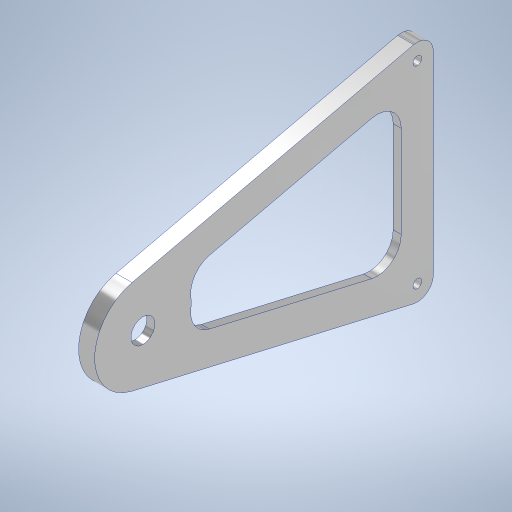
# Autodesk Inventor part: Frame (Motor Side)
Saved by Autodesk Inventor 2023.2 (Build 272271000, 271)
## iProperties
Created: 2022-05-22
Part Number: Frame (Motor Side)
Material: Aluminum 6061
Document SubType Name: Modeling
Designer: Nathan Cai
Density: 2.7 g/cm^3
Appearance: Aluminum - Flat
Mass: 63.0203 g
Surface Area: 136.097 cm^2
Volume: 23.3409 cm^3
Leg_Mounts: 0.625 in
Leg_Offset: 0.750 in
C2C: 4.265 in
Author: Nathan Cai
Autodesk Inventor part; units mm, degrees
ref_plane "YZ Plane" through (0, 0, 0) normal (1, 0, 0) x (0, 1, 0)
ref_plane "XZ Plane" through (0, 0, 0) normal (0, 1, 0) x (-1, 0, 0)
ref_plane "XY Plane" through (0, 0, 0) normal (0, 0, 1) x (1, 0, 0)
sketch "Sketch1" plane through (0, 0, 0) normal (1, 0, 0) x (0, 1, 0)
  circle A0 centre (0, 0) radius 4.7625 construction
  line L0 (0, 0) -> (0, 108.331) construction
  circle A1 centre (0, 108.331) radius 4.7625
  circle A2 centre (0, 108.331) radius 76.2 construction
  circle A3 centre (0, 108.331) radius 19.05
  line L1 (0, 0) -> (38.1, 0) construction
  circle A4 centre (38.1, 0) radius 1.7526
  circle A5 centre (38.1, 0) radius 6.35
  line L2 (18.5597, 112.6252) -> (44.2866, 1.4314)
  line L3 (10.2351, 92.2641) -> (31.9134, -1.4314)
  circle A6 centre (-38.1, 0) radius 1.7526
  circle A7 centre (-38.1, 0) radius 6.35
  line L4 (-18.5597, 112.6252) -> (-44.2866, 1.4314)
  line L5 (-10.2351, 92.2641) -> (-31.9134, -1.4314)
  line L6 (38.1, 6.35) -> (-38.1, 6.35)
  line L7 (-38.1, -6.35) -> (38.1, -6.35)
  line L8 (38.1, 0) -> (15.5738, 97.3602) construction
  circle A8 centre (19.05, 82.3358) radius 1.7526
  circle A9 centre (-19.05, 82.3358) radius 1.7526
  line L9 (19.05, 82.3358) -> (-19.05, 82.3358) construction
  circle A10 centre (15.875, 82.3358) radius 6.35
  circle A11 centre (15.875, 82.3358) radius 1.7526
  circle A12 centre (-15.875, 82.3358) radius 6.35
  circle A13 centre (-15.875, 82.3358) radius 1.7526
  arc A14 (31.7424, -0.6924) -> (-31.1085, -6.35) centre (0, 0) ccw construction
  arc A15 (44.45, 0) -> (-44.45, 0) centre (0, 0) ccw construction
  point P0 (44.2067, -1.741)
  point P1 (-22.5544, 39.0194)
  point P2 (-10.2351, 92.2641)
  point P3 (30.1131, 6.35)
  point P4 (-30.1131, 6.35)
  point P5 (-13.9309, 76.2907)
  point P6 (-11.4733, 86.9126)
  point P7 (11.4733, 86.9126)
  point P8 (13.9309, 76.2907)
  point P9 (22.7465, 38.189)
  point P10 (-22.7465, 38.189)
  point P11 (-40.2576, 18.8447)
  point P12 (-44.3636, 7.3939)
  point P13 (-31.75, 0)
  point P14 (31.75, 0)
  point P15 (44.3636, 7.3939)
  point P16 (40.2576, 18.8447)
  point P17 (-28.2125, 14.5642)
  point P18 (31.8736, 5.0775)
  point P19 (-31.7424, -0.6924)
  point P20 (28.2125, 14.5642)
  dimension "d0" = 9.525
  dimension "C2C" = 108.331
  dimension "d3" = 9.525
  dimension "d4" = 152.4
  dimension "d5" = 38.1
  dimension "d6" = 38.1
  dimension "d7" = 3.5052
  dimension "d8" = 12.7
  dimension "d9" = 0
  dimension "d10" = 12.7
  dimension "d37" = 3.5052
  dimension "Leg_Offset" = 19.05
  dimension "d39" = 12.7
  dimension "d40" = 3.5052
  dimension "Leg_Mounts" = 15.875
  dimension "d42" = 12.7
  constraints: 20 end point, 18 point on circle, 16 centre point, 11 coincident, 10 symmetric about line, 7 tangent, 6 point on line, 2 horizontal, 2 parallel, 1 vertical, 5 other
  measures "d0" diameter of A0
  measures "C2C" distance of L0.start L0.end
  measures "d3" diameter of A1
  measures "d4" diameter of A2
  measures "d5" diameter of A3
  measures "d6" distance of L1.start L1.end
  measures "d7" diameter of A4
  measures "d8" diameter of A5
  measures "d9" distance from line of A0.centre L1
  measures "d10" distance between parallel lines of L2 L3
  measures "d37" diameter of A8
  measures "Leg_Offset" distance from line of L0 L9.start
  measures "d39" diameter of A10
  measures "d40" diameter of A11
  measures "Leg_Mounts" distance from line of L0 A11.centre
  measures "d42" radial gap between concentric circles of A14 A15
extrude "Extrusion1" add sketch "Sketch1" along normal blind 6.35 contours A3 | A3 L2 A5 L6 L3 A10 | A3 L5 A12 L6 A7 L4 | A5 | A10 L3 | A7 | A5 L3 L6 | L5 A12 | L6 L5 A7 | A7 L5 L6 L3 A5 L7 | A8 A11 | A11 A8 | A8 A11 | A9 A13 | A9 A13 | A13 A9 picked at (13.1931, 81.7042) picked at (-13.1931, 81.7042)
fillet "Fillet1" radius 9.525 4 edges at (3.175, 10.2351, 92.2641) (3.175, -10.2351, 92.2641) (3.175, 30.1131, 6.35) (3.175, -30.1131, 6.35)
sketch "Sketch2" plane through (0, 0, 0) normal (1, 0, 0) x (0, 0, -1)
  line L0 (-1.4314, 44.2866) -> (-112.6252, 18.5597) projected
  circle A0 centre (0, 38.1) radius 6.35
  circle A1 centre (0, -38.1) radius 1.7526 projected
  arc A2 (-1.4314, -44.2866) -> (6.35, -38.1) centre (0, -38.1) ccw projected
  circle A3 centre (0, -38.1) radius 6.35
  circle A4 centre (0, 38.1) radius 1.7526 projected
  line L1 (-18.0221, -27.4125) -> (-82.0952, -12.5879) projected
  circle A5 centre (0, -38.1) radius 1.7526 projected
  circle A6 centre (-108.331, 0) radius 4.7625 projected
  circle A7 centre (0, 38.1) radius 1.7526 projected
  line L2 (6.35, -38.1) -> (6.35, 38.1) projected
  arc A8 (6.35, 38.1) -> (-1.4314, 44.2866) centre (0, 38.1) ccw projected
  line L3 (-1.4314, 44.2866) -> (-112.6252, 18.5597) projected
  line L4 (-112.6252, -18.5597) -> (-1.4314, -44.2866) projected
  arc A9 (-1.4314, -44.2866) -> (6.35, -38.1) centre (0, -38.1) ccw projected
  line L5 (-18.0221, -27.4125) -> (-82.0952, -12.5879) projected
  circle A10 centre (0, -38.1) radius 1.7526 projected
  circle A11 centre (-108.331, 0) radius 4.7625 projected
  circle A12 centre (0, 38.1) radius 1.7526 projected
  line L6 (6.35, -38.1) -> (6.35, 38.1) projected
  arc A13 (6.35, 38.1) -> (-1.4314, 44.2866) centre (0, 38.1) ccw projected
  line L7 (-1.4314, 44.2866) -> (-112.6252, 18.5597) projected
  line L8 (-112.6252, -18.5597) -> (-1.4314, -44.2866) projected
  arc A14 (-1.4314, -44.2866) -> (6.35, -38.1) centre (0, -38.1) ccw projected
  line L9 (-82.0952, 12.5879) -> (-18.0221, 27.4125) projected
  arc A15 (-6.35, 18.1326) -> (-18.0221, 27.4125) centre (-15.875, 18.1326) ccw projected
  line L10 (-6.35, 18.1326) -> (-6.35, -18.1326) projected
  arc A16 (-18.0221, -27.4125) -> (-6.35, -18.1326) centre (-15.875, -18.1326) ccw projected
  line L11 (-82.0952, 12.5879) -> (-18.0221, 27.4125) projected
  arc A17 (-6.35, 18.1326) -> (-18.0221, 27.4125) centre (-15.875, 18.1326) ccw projected
  line L12 (-6.35, 18.1326) -> (-6.35, -18.1326) projected
  arc A18 (-18.0221, -27.4125) -> (-6.35, -18.1326) centre (-15.875, -18.1326) ccw projected
  arc A19 (-89.4091, -2.2054) -> (-82.0952, -12.5879) centre (-79.9481, -3.3081) ccw projected
  arc A20 (-89.4091, -2.2054) -> (-89.4091, 2.2054) centre (-108.331, 0) ccw projected
  arc A21 (-82.0952, 12.5879) -> (-89.4091, 2.2054) centre (-79.9481, 3.3081) ccw projected
  arc A22 (-112.6252, 18.5597) -> (-112.6252, -18.5597) centre (-108.331, 0) ccw projected
  arc A23 (-89.4091, -2.2054) -> (-82.0952, -12.5879) centre (-79.9481, -3.3081) ccw projected
  arc A24 (-89.4091, -2.2054) -> (-89.4091, 2.2054) centre (-108.331, 0) ccw projected
  arc A25 (-82.0952, 12.5879) -> (-89.4091, 2.2054) centre (-79.9481, 3.3081) ccw projected
  arc A26 (-112.6252, 18.5597) -> (-112.6252, -18.5597) centre (-108.331, 0) ccw projected
  line L13 (-1.4314, 44.2866) -> (-112.6252, 18.5597) projected
  arc A27 (6.35, 38.1) -> (-1.4314, 44.2866) centre (0, 38.1) ccw projected
  line L14 (6.35, -38.1) -> (6.35, 38.1) projected
  arc A28 (-1.4314, -44.2866) -> (6.35, -38.1) centre (0, -38.1) ccw projected
  line L15 (-112.6252, -18.5597) -> (-1.4314, -44.2866) projected
  arc A29 (-112.6252, 18.5597) -> (-112.6252, -18.5597) centre (-108.331, 0) ccw projected
  circle A30 centre (-108.331, 0) radius 4.7625 projected
  circle A31 centre (0, 38.1) radius 1.7526 projected
  circle A32 centre (0, -38.1) radius 1.7526 projected
  arc A33 (-6.35, 18.1326) -> (-18.0221, 27.4125) centre (-15.875, 18.1326) ccw projected
  line L16 (-82.0952, 12.5879) -> (-18.0221, 27.4125) projected
  arc A34 (-82.0952, 12.5879) -> (-89.4091, 2.2054) centre (-79.9481, 3.3081) ccw projected
  arc A35 (-89.4091, -2.2054) -> (-89.4091, 2.2054) centre (-108.331, 0) ccw projected
  arc A36 (-89.4091, -2.2054) -> (-82.0952, -12.5879) centre (-79.9481, -3.3081) ccw projected
  line L17 (-18.0221, -27.4125) -> (-82.0952, -12.5879) projected
  arc A37 (-18.0221, -27.4125) -> (-6.35, -18.1326) centre (-15.875, -18.1326) ccw projected
  line L18 (-6.35, 18.1326) -> (-6.35, -18.1326) projected
  line L19 (-6.1866, -36.6686) -> (-83.5266, -18.7745)
  arc A38 (-95.7164, -1.4702) -> (-83.5266, -18.7745) centre (-79.9481, -3.3081) ccw
  arc A39 (-95.7164, -1.4702) -> (-95.7164, 1.4702) centre (-108.331, 0) ccw
  arc A40 (-83.5266, 18.7745) -> (-95.7164, 1.4702) centre (-79.9481, 3.3081) ccw
  line L20 (-83.5266, 18.7745) -> (-6.1866, 36.6686)
  circle A41 centre (-108.331, 0) radius 11.1125
  arc A42 (-89.4091, -2.2054) -> (-89.4091, 2.2054) centre (-108.331, 0) ccw projected
  line L21 (-108.331, 0) -> (6.35, 0) construction
  point P0 (6.35, -38.1)
  point P1 (6.35, 38.1)
  point P2 (6.35, 38.1)
  point P3 (6.35, 38.1)
  dimension "d66" = 6.35
  dimension "d67" = 22.225
  dimension "d68" = 6.35
  dimension "d69" = 6.35
  constraints: 10 point on circle, 6 centre point, 6 end point, 3 coincident, 2 parallel, 1 midpoint, 2 other
  measures "d66" distance between parallel lines of L1 L19
  measures "d67" diameter of A41
  measures "d68" radial gap between concentric circles of A19 A38
  measures "d69" radial gap between concentric circles of A20 A39
extrude "Extrusion4" cut sketch "Sketch2" along normal blind 3.175 contours L2 A3 L19 A38 A39 A40 L20 A0
extrude "Extrusion5" cut sketch "Sketch2" along normal blind 3.175 contours A41
fillet "Fillet4" radius 6.35 2 edges at (1.5875, -36.6686, 6.1866) (1.5875, 36.6686, 6.1866)
equation "\"d10\" = d8"
body "Solid1"
